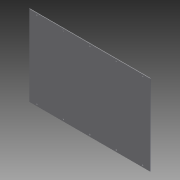
# Autodesk Inventor part: top
Saved by Autodesk Inventor 2012 (Build 160160000, 160)
## iProperties
Created: 2012-05-13
Part Number: top
Material: Default
Document SubType Name: Modeling
Designer: Puzzles
Density: 1 g/cm^3
Author: Puzzles
Autodesk Inventor part; units mm, degrees
ref_plane "YZ Plane" through (0, 0, 0) normal (1, 0, 0) x (0, 1, 0)
ref_plane "XZ Plane" through (0, 0, 0) normal (0, 1, 0) x (-1, 0, 0)
ref_plane "XY Plane" through (0, 0, 0) normal (0, 0, 1) x (1, 0, 0)
sketch "Sketch1" plane through (0, 0, 0) normal (0, 0, 1) x (1, 0, 0)
  line L0 (-304.8, 203.2) -> (304.8, 203.2)
  line L1 (304.8, 203.2) -> (304.8, -203.2)
  line L2 (304.8, -203.2) -> (-304.8, -203.2)
  line L3 (-304.8, -203.2) -> (-304.8, 203.2)
  point P0 (0, 0)
  point P1 (0, 203.2)
  point P2 (304.8, 0)
  dimension "d0" = 609.6
  dimension "d1" = 406.4
  constraints: 8 end point, 2 midpoint, 2 parallel, 1 horizontal, 1 horizontal alignment, 1 perpendicular, 1 vertical alignment
  measures "d0" distance of L0.start L0.end
  measures "d1" distance of L2.end L0.start
extrude "Extrusion1" add sketch "Sketch1" along normal blind 3
sketch "Sketch2" plane through (0, 0, 3) normal (0, 0, 1) x (1, 0, 0)
  line L0 (304.8, 203.2) -> (304.8, -203.2) projected
  line L1 (-304.8, -203.2) -> (-304.8, 203.2) projected
  line L2 (304.8, -203.2) -> (-304.8, -203.2) projected
  line L3 (-304.8, 0) -> (304.8, 0)
  point P0 (0, 0)
  point P1 (-266.7, -193.675)
  point P2 (-133.35, -193.675)
  point P3 (0, -193.675)
  point P4 (133.35, -193.675)
  point P5 (266.7, -193.675)
  point P6 (-266.7, 193.675)
  point P7 (-133.35, 193.675)
  point P8 (0, 193.675)
  point P9 (133.35, 193.675)
  point P10 (266.7, 193.675)
  dimension "d4" = 9.525
  dimension "d5" = 133.35
  dimension "d6" = 38.1
  dimension "d7" = 133.35
  dimension "d8" = 133.35
  dimension "d9" = 133.35
  dimension "d10" = 38.1
  constraints: 5 symmetric about line, 2 end point, 2 midpoint
  measures "d4" distance from line of point (-266.7, -193.675) L2
  measures "d5" distance of point (-266.7, -193.675) point (-133.35, -193.675)
  measures "d6" distance from line of L1 point (-266.7, -193.675)
  measures "d7" distance of point (-133.35, -193.675) point (0, -193.675)
  measures "d8" distance of point (0, -193.675) point (133.35, -193.675)
  measures "d9" distance of point (133.35, -193.675) point (266.7, -193.675)
  measures "d10" distance from line of L0 point (266.7, -193.675)
hole "Hole1" at (-266.7, -193.675, 3) at (-133.35, -193.675, 3) at (0, -193.675, 3) at (133.35, -193.675, 3) at (266.7, -193.675, 3) at (-266.7, 193.675, 3) at (-133.35, 193.675, 3) at (0, 193.675, 3) at (133.35, 193.675, 3) at (266.7, 193.675, 3) direction (0, 0, -1) diameter 6.35 end through all
body "Solid1"
